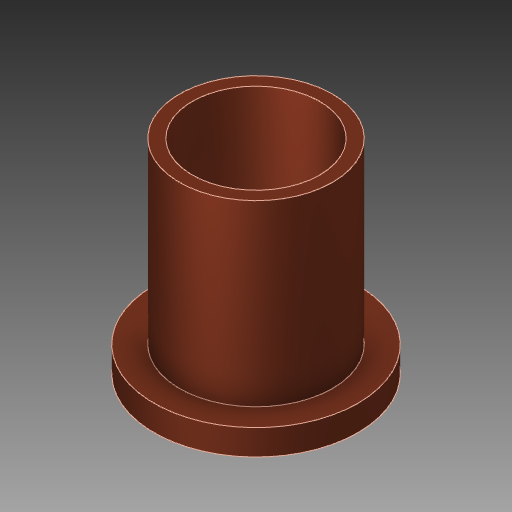
# Autodesk Inventor part: 6338K471
Saved by Autodesk Inventor 2023 (Build 270158030, 158C)
## iProperties
Created: 2020-11-18
Part Number: 6338K471
Material: Bronze, Cast
Document SubType Name: Modeling
Density: 8.87 g/cm^3
Appearance: Copper - Satin
Mass: 37.9047 g
Surface Area: 56.5296 cm^2
Volume: 4.27337 cm^3
Revision Number: 0
Autodesk Inventor part; units mm, degrees
ref_plane "YZ Plane" through (0, 0, 0) normal (1, 0, 0) x (0, 1, 0)
ref_plane "XZ Plane" through (0, 0, 0) normal (0, 1, 0) x (-1, 0, 0)
ref_plane "XY Plane" through (0, 0, 0) normal (0, 0, 1) x (1, 0, 0)
sketch "Sketch1" plane through (0, 0, 0) normal (0, 0, 1) x (1, 0, 0)
  line L0 (0, 0) -> (0, 12.7) construction
  line L1 (7.9375, 12.7) -> (7.9375, -12.7)
  line L2 (7.9375, 12.7) -> (0, 0) construction
  line L3 (7.9375, -12.7) -> (0, 0) construction
  line L4 (7.9375, 12.7) -> (9.525, 12.7)
  line L5 (9.525, 12.7) -> (9.525, -9.525)
  line L6 (9.525, -9.525) -> (12.7, -9.525)
  line L7 (12.7, -9.525) -> (12.7, -12.7)
  line L8 (12.7, -12.7) -> (7.9375, -12.7)
  dimension "ID" = 15.875
  dimension "OD" = 19.05
  dimension "Thickness" = 3.175
  dimension "FlangeOD" = 25.4
  dimension "length" = 25.4
  constraints: 18 end point, 4 perpendicular, 2 vertical, 1 equal length, 1 horizontal, 1 horizontal alignment
  measures "ID" diameter of L1 L0
  measures "OD" diameter of L5 L0
  measures "Thickness" distance between parallel lines of L8 L6
  measures "FlangeOD" diameter of L7 L0
  measures "length" distance between parallel lines of L8 L4
revolve "Revolution1" add sketch "Sketch1" angle 360 about axis through (0, 0, 0) along (0, 1, 0)
body "Solid1"
